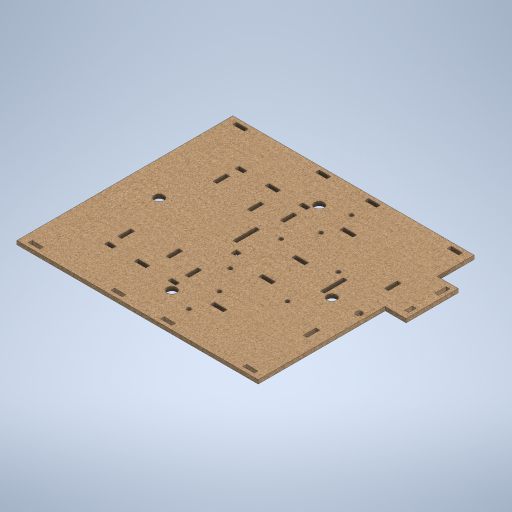
# Autodesk Inventor part: Base3
Saved by Autodesk Inventor 2024 (Build 280153000, 153)
## iProperties
Created: 2023-11-22
Part Number: Base3
Material: MDF Tablero de fibras de densidad media
Document SubType Name: Modeling
Designer: marco
Density: 0.8 g/cm^3
Appearance: Cartón - Ondulado
Author: marco
Autodesk Inventor part; units mm, degrees
ref_plane "YZ Plane" through (0, 0, 0) normal (1, 0, 0) x (0, 1, 0)
ref_plane "XZ Plane" through (0, 0, 0) normal (0, 1, 0) x (-1, 0, 0)
ref_plane "XY Plane" through (0, 0, 0) normal (0, 0, 1) x (1, 0, 0)
sketch "Boceto1" plane through (0, 0, 0) normal (0, 1, 0) x (-1, 0, 0)
  circle A0 centre (-19.5, -64) radius 1.5
  circle A1 centre (-19.5, -40) radius 1.5
  circle A2 centre (0, 58) radius 3.75
  circle A3 centre (-19.5, 40) radius 1.5
  circle A4 centre (-19.5, 64) radius 1.5
  line L0 (37, -85) -> (-95, -85)
  circle A5 centre (-89.5, 0) radius 2.5
  circle A6 centre (-53.0625, 20) radius 1.5
  circle A7 centre (-53.0625, -20) radius 1.5
  circle A8 centre (-8.0625, -20) radius 1.5
  circle A9 centre (-8.0625, 20) radius 1.5
  line L1 (15, 82) -> (15, 79)
  line L2 (24, 79) -> (24, 82)
  line L3 (-89, -79) -> (-89, -82)
  line L4 (-80, -82) -> (-80, -79)
  line L5 (-15, -85) -> (-95, -85)
  line L6 (-15, -82) -> (-15, -79)
  line L7 (15, -79) -> (15, -82)
  circle A10 centre (-68, 0) radius 3.75
  circle A11 centre (0, -58) radius 3.75
  line L8 (24, -82) -> (24, -79)
  line L9 (89, -79) -> (89, -82)
  circle A12 centre (68, 0) radius 3.75
  line L10 (-89, 82) -> (-89, 79)
  line L11 (-80, 79) -> (-80, 82)
  line L12 (89, 79) -> (89, 82)
  line L13 (95, 15) -> (95, 85)
  line L14 (-15, 85) -> (-95, 85)
  line L15 (55, 42.5) -> (58, 42.5)
  line L16 (58, 42.5) -> (58, 32.5)
  line L17 (58, 32.5) -> (55, 32.5)
  line L18 (15, 79) -> (24, 79)
  line L19 (24, 79) -> (24, 82)
  line L20 (24, 82) -> (15, 82)
  line L21 (-89, -82) -> (-80, -82)
  line L22 (-80, -82) -> (-80, -79)
  line L23 (-80, -79) -> (-89, -79)
  line L24 (-15, -82) -> (-24, -82)
  line L25 (-24, -82) -> (-24, -79)
  line L26 (-24, -79) -> (-15, -79)
  line L27 (15, -82) -> (24, -82)
  line L28 (24, -82) -> (24, -79)
  line L29 (24, -79) -> (15, -79)
  line L30 (-89, 79) -> (-80, 79)
  line L31 (-80, 79) -> (-80, 82)
  line L32 (-80, 82) -> (-89, 82)
  line L33 (-15, 82) -> (-24, 82)
  line L34 (-24, 82) -> (-24, 79)
  line L35 (-24, 79) -> (-15, 79)
  line L36 (-15, 79) -> (-15, 82)
  line L37 (25.5, 27) -> (25.5, 37)
  line L38 (25.5, 37) -> (22.5, 37)
  line L39 (22.5, 37) -> (22.5, 27)
  line L40 (22.5, 27) -> (25.5, 27)
  line L41 (22.5, -27) -> (25.5, -27)
  line L42 (25.5, -27) -> (25.5, -37)
  line L43 (25.5, -37) -> (22.5, -37)
  line L44 (22.5, -37) -> (22.5, -27)
  line L45 (-25, -49.5) -> (-25, -52.5)
  line L46 (-25, -52.5) -> (-35, -52.5)
  line L47 (-35, -52.5) -> (-35, -49.5)
  line L48 (-35, -49.5) -> (-25, -49.5)
  line L49 (-35, -14.5) -> (-25, -14.5)
  line L50 (-25, -14.5) -> (-25, -11.5)
  line L51 (-25, -11.5) -> (-35, -11.5)
  line L52 (-35, -11.5) -> (-35, -14.5)
  line L53 (-35, 11.5) -> (-25, 11.5)
  line L54 (-25, 11.5) -> (-25, 14.5)
  line L55 (-25, 14.5) -> (-35, 14.5)
  line L56 (-35, 14.5) -> (-35, 11.5)
  line L57 (-35, 52.5) -> (-35, 49.5)
  line L58 (-35, 49.5) -> (-25, 49.5)
  line L59 (-25, 49.5) -> (-25, 52.5)
  line L60 (-25, 52.5) -> (-35, 52.5)
  line L61 (-85.5, 27) -> (-82.5, 27)
  line L62 (-82.5, 27) -> (-82.5, 37)
  line L63 (-82.5, 37) -> (-85.5, 37)
  line L64 (-85.5, 37) -> (-85.5, 27)
  line L65 (-82.5, -27) -> (-82.5, -37)
  line L66 (-82.5, -37) -> (-85.5, -37)
  line L67 (-85.5, -37) -> (-85.5, -27)
  line L68 (-85.5, -27) -> (-82.5, -27)
  line L69 (52, -50) -> (58, -50)
  line L70 (58, -50) -> (58, -53)
  line L71 (58, -53) -> (55, -53)
  line L72 (55, -53) -> (52, -53)
  line L73 (52, -53) -> (52, -50)
  line L74 (2, -53) -> (8, -53)
  line L75 (8, -53) -> (8, -50)
  line L76 (8, -50) -> (2, -50)
  line L77 (2, -50) -> (2, -53)
  line L78 (2, 53) -> (8, 53)
  line L79 (8, 53) -> (8, 50)
  line L80 (8, 50) -> (2, 50)
  line L81 (2, 50) -> (2, 53)
  line L82 (55, 50) -> (58, 50)
  line L83 (58, 50) -> (58, 53)
  line L84 (58, 53) -> (52, 53)
  line L85 (52, 53) -> (52, 50)
  line L86 (52, 50) -> (55, 50)
  line L87 (34.5, 53) -> (34.5, 50)
  line L88 (34.5, 50) -> (25.5, 50)
  line L89 (25.5, 50) -> (25.5, 53)
  line L90 (25.5, 53) -> (34.5, 53)
  line L91 (34.5, -50) -> (34.5, -53)
  line L92 (34.5, -53) -> (25.5, -53)
  line L93 (25.5, -53) -> (25.5, -50)
  line L94 (25.5, -50) -> (34.5, -50)
  line L95 (55, 42.5) -> (55, 32.5)
  line L96 (55, 32.5) -> (58, 32.5)
  line L97 (58, 32.5) -> (58, 42.5)
  line L98 (58, 42.5) -> (55, 42.5)
  line L99 (5, 32.5) -> (2, 32.5)
  line L100 (2, 32.5) -> (2, 42.5)
  line L101 (2, 42.5) -> (5, 42.5)
  line L102 (5, 42.5) -> (5, 32.5)
  line L103 (58, 42.5) -> (55, 42.5)
  line L104 (55, 42.5) -> (55, 32.5)
  line L105 (55, 32.5) -> (58, 32.5)
  line L106 (58, 32.5) -> (58, 42.5)
  line L107 (5, -32.5) -> (2, -32.5)
  line L108 (2, -32.5) -> (2, -42.5)
  line L109 (2, -42.5) -> (5, -42.5)
  line L110 (5, -42.5) -> (5, -32.5)
  line L111 (58, -42.5) -> (55, -42.5)
  line L112 (55, -42.5) -> (55, -32.5)
  line L113 (55, -32.5) -> (58, -32.5)
  line L114 (58, -32.5) -> (58, -42.5)
  line L115 (-62.125, -18) -> (-59.125, -18)
  line L116 (-59.125, -18) -> (-59.125, 0)
  line L117 (-59.125, 0) -> (-62.125, 0)
  line L118 (-62.125, 0) -> (-62.125, -18)
  line L119 (-2, 9.25) -> (2, 9.25)
  line L120 (2, 9.25) -> (2, 5.25)
  line L121 (2, 5.25) -> (-2, 5.25)
  line L122 (-2, 5.25) -> (-2, 9.25)
  line L123 (6.875, 0) -> (6.875, -18)
  line L124 (6.875, -18) -> (9.875, -18)
  line L125 (9.875, -18) -> (9.875, 0)
  line L126 (9.875, 0) -> (6.875, 0)
  line L127 (80, 79) -> (80, 82)
  line L128 (80, 82) -> (89, 82)
  line L129 (89, 82) -> (89, 79)
  line L130 (89, 79) -> (80, 79)
  line L131 (80, -79) -> (89, -79)
  line L132 (89, -79) -> (89, -82)
  line L133 (89, -82) -> (80, -82)
  line L134 (80, -82) -> (80, -79)
  line L135 (-95, -56) -> (-95, -85)
  line L136 (-95, -85) -> (95, -85)
  line L137 (95, -85) -> (95, 85)
  line L138 (95, 85) -> (-95, 85)
  line L139 (-95, 85) -> (-95, -15)
  line L140 (-95, -15) -> (-111.5, -15)
  line L141 (-111.5, -15) -> (-111.5, -56)
  line L142 (-111.5, -56) -> (-95, -56)
  line L143 (95, -85) -> (95, 85)
  line L144 (95, 85) -> (-95, 85)
  line L145 (-95, 85) -> (-95, -15)
  line L146 (-95, -15) -> (-111.5, -15)
  line L147 (-111.5, -15) -> (-111.5, -56)
  line L148 (-111.5, -56) -> (-95, -56)
  line L149 (-95, -56) -> (-95, -85)
  line L150 (-95, -85) -> (95, -85)
  line L151 (-108.5, -43.5) -> (-105.5, -43.5)
  line L152 (-105.5, -43.5) -> (-105.5, -52.5)
  line L153 (-105.5, -52.5) -> (-108.5, -52.5)
  line L154 (-108.5, -52.5) -> (-108.5, -43.5)
  line L155 (-108.5, -26) -> (-108.5, -20)
  line L156 (-108.5, -20) -> (-105.5, -20)
  line L157 (-105.5, -20) -> (-105.5, -26)
  line L158 (-105.5, -26) -> (-108.5, -26)
  point P0 (0, 0)
  point P1 (2, -32.5)
  point P2 (2, 32.5)
  point P3 (2, 50)
  point P4 (2, -50)
  constraints: 318 end point, 13 centre point
extrude "Extrusión1" add sketch "Boceto1" along normal blind 3
